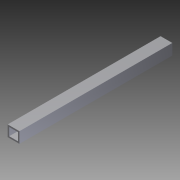
# Autodesk Inventor part: InternalBar
Saved by Autodesk Inventor 2012 (Build 160160000, 160)
## iProperties
Created: 2012-01-12
Part Number: InternalBar
Material: Default
Document SubType Name: Modeling
Designer: William
Density: 1 g/cm^3
Author: William
Autodesk Inventor part; units mm, degrees
ref_plane "YZ Plane" through (0, 0, 0) normal (1, 0, 0) x (0, 1, 0)
ref_plane "XZ Plane" through (0, 0, 0) normal (0, 1, 0) x (-1, 0, 0)
ref_plane "XY Plane" through (0, 0, 0) normal (0, 0, 1) x (1, 0, 0)
sketch "Sketch1" plane through (0, 0, 0) normal (0, 0, 1) x (1, 0, 0)
  line L0 (3.9902, -4.7999) -> (-15.0598, -4.7999)
  line L1 (-15.0598, -4.7999) -> (-15.0598, 12.506)
  line L2 (-15.0598, 12.506) -> (3.9902, 12.506)
  line L3 (3.9902, 12.506) -> (3.9902, -4.7999)
  line L4 (-18.2348, 15.681) -> (7.1652, 15.681)
  line L5 (7.1652, 15.681) -> (7.1652, -7.9749)
  line L6 (7.1652, -7.9749) -> (-18.2348, -7.9749)
  line L7 (-18.2348, -7.9749) -> (-18.2348, 15.681)
  point P0 (0, 0)
  dimension "d0" = 25.4
  dimension "d1" = 23.6559
  dimension "d2" = 3.175
  dimension "d3" = 3.175
  dimension "d4" = 3.175
  dimension "d5" = 3.175
  constraints: 16 end point, 4 parallel, 2 horizontal, 2 perpendicular
  measures "d0" distance of L4.start L4.end
  measures "d1" distance of L6.end L4.start
  measures "d2" distance between parallel lines of L7 L1
  measures "d3" distance between parallel lines of L4 L2
  measures "d4" distance between parallel lines of L6 L0
  measures "d5" distance between parallel lines of L5 L3
extrude "Extrusion1" add sketch "Sketch1" along normal blind 330.2
equation "\"d3\" = d2"
equation "\"d4\" = d3"
equation "\"d5\" = d4"
body "Solid1"
